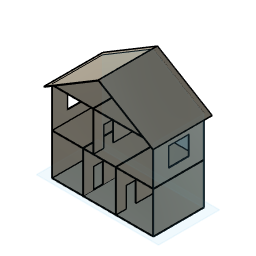
model (Autodesk Fusion 360 design; units mm, degrees)
Autodesk Fusion 360 part; units mm, degrees
note: some values were not read from the file. Set by a fixed rule: which sketch regions a step uses.
sketch "Sketch1" plane through (0, 0, 0) normal (0, 0, 1) x (1, 0, 0)
  line L0 (-300, 150) -> (300, 150)
  line L1 (300, 150) -> (300, -150)
  line L2 (300, -150) -> (-300, -150)
  line L3 (-300, -150) -> (-300, 150)
  line L4 (-300, 0) -> (300, 0) construction
  dimension "d4" = 600
  dimension "d5" = 300
  constraint horizontal L0
  constraint vertical L1
  constraint horizontal L2
  constraint vertical L3
  constraint midpoint L3 L4.start
  constraint midpoint L1 L4.end
  constraint midpoint origin L4
  measures "d4" distance of L0.start L0.end
  measures "d5" distance of L0.start L2.end
sketch "Sketch2" plane through (0, 0, 0) normal (0, 0, -1) x (1, 0, 0)
  line L0 (300, 150) -> (-300, 150)
  line L1 (-300, 150) -> (-300, -150)
  line L2 (-300, -150) -> (300, -150)
  line L3 (300, -150) -> (300, 150)
  line L4 (-250, 125) -> (-247, 125)
  line L5 (-247, 125) -> (-247, -125)
  line L6 (-247, -125) -> (-250, -125)
  line L7 (-250, -125) -> (-250, 125)
  line L8 (250, 125) -> (247, 125)
  line L9 (247, 125) -> (247, -125)
  line L10 (247, -125) -> (250, -125)
  line L11 (250, -125) -> (250, 125)
  dimension "d8" = 3
  dimension "d9" = 3
  dimension "d10" = 50
  dimension "d11" = 50
  dimension "d12" = 25
  dimension "d13" = 25
  dimension "d14" = 25
  dimension "d15" = 25
  constraint horizontal L4
  constraint vertical L5
  constraint horizontal L6
  constraint vertical L7
  constraint horizontal L8
  constraint vertical L9
  constraint horizontal L10
  constraint vertical L11
  measures "d8" distance of L5 L7
  measures "d9" distance of L9 L11
  measures "d10" distance of L3 L11
  measures "d11" distance of L1 L7
  measures "d12" distance of L0 L4.start
  measures "d13" distance of L0 L8.start
  measures "d14" distance of L2 L9.end
  measures "d15" distance of L2 L5.end
extrude "Extrude2" add sketch "Sketch2" against normal blind 400 contours L4 L5 L6 L7 | L8 L9 L10 L11 makes body 1 at (-247, -41.6667, 133.3333) makes body 2 at (250, 41.6667, 133.3333)
sketch "Sketch3" plane through (0, 0, 0) normal (0, 0, -1) x (1, 0, 0)
  line L0 (300, 150) -> (-300, 150)
  line L1 (-300, 150) -> (-300, -150)
  line L2 (-300, -150) -> (300, -150)
  line L3 (300, -150) -> (300, 150)
  line L4 (-250, -125) -> (-250, 125)
  line L5 (250, -125) -> (250, 125)
  line L6 (-250, -125) -> (250, -125)
  line L7 (250, -125) -> (250, -122)
  line L8 (250, -122) -> (-250, -122)
  line L9 (-250, -122) -> (-250, -125)
  dimension "d18" = 3
  constraint horizontal L6
  constraint vertical L7
  constraint horizontal L8
  constraint vertical L9
  constraint coincident L5 L7.end
  constraint coincident L4.start L6.start
  measures "d18" distance of L6 L8
extrude "Extrude3" add sketch "Sketch3" against normal blind 400 separate body contours L4 L5 L6 L7 L8 L9 makes body 3
sketch "Sketch4" plane through (0, 125, 0) normal (0, 1, 0) x (-1, 0, 0)
  line L0 (-250, 0) -> (250, 0)
  line L1 (250, 0) -> (250, 400)
  line L2 (250, 400) -> (-250, 400)
  line L3 (-250, 400) -> (-250, 0)
  line L4 (-250, 400) -> (0, 550)
  line L5 (0, 550) -> (250, 400)
  line L6 (0, 550) -> (0, 400) construction
  dimension "d21" = 150
  constraint coincident L2.end L3.start
  constraint coincident L1.end L2.start
  constraint midpoint L2 L6.end
  constraint perpendicular L2 L6
  measures "d21" distance of L4.end L6.end
extrude "Extrude4" add sketch "Sketch4" against normal blind 3 separate body contours L2 L4 L5 makes body 4
combine "Combine1" operation add target body 3 tool bodies 4
sketch "Sketch5" plane through (242.6471, 0, 404.4118) normal (0.514496, 0, 0.857493) x (0, 1, 0)
  line L0 (125, -8.5749) -> (125, 282.9727)
  line L1 (125, 282.9727) -> (122, 282.9727)
  line L2 (122, 282.9727) -> (122, -8.5749)
  line L3 (122, -8.5749) -> (125, -8.5749)
  line L4 (145, 285.9727) -> (-145, 285.9727)
  line L5 (-145, 285.9727) -> (-145, -28.5749)
  line L6 (-145, -28.5749) -> (145, -28.5749)
  line L7 (145, -28.5749) -> (145, 285.9727)
  line L8 (-125, -214.3732) -> (-125, -8.5749)
  line L9 (-125, -8.5749) -> (125, -8.5749)
  dimension "d24" = 20
  dimension "d25" = 20
  dimension "d26" = 3
  dimension "d27" = 20
  constraint horizontal L4
  constraint vertical L5
  constraint horizontal L6
  constraint vertical L7
  measures "d24" distance of L0 L6.end
  measures "d25" distance of L5 L8
  measures "d26" distance of L1.end L4
  measures "d27" distance of L6 L9
extrude "Extrude5" add sketch "Sketch5" along normal blind 3 separate body contours L0 L1 L2 L3 L9 | L4 L5 L6 L7 makes body 5
sketch "Sketch6" plane through (-242.6471, 0, 404.4118) normal (-0.514496, 0, 0.857493) x (0, -1, 0)
  line L0 (-125, 282.9727) -> (-125, -8.5749)
  line L1 (-125, -8.5749) -> (-122, -8.5749)
  line L2 (-122, -8.5749) -> (-122, 282.9727)
  line L3 (-122, 282.9727) -> (-125, 282.9727)
  line L4 (-145, 281.5609) -> (145, 281.5609)
  line L5 (-145, 281.5609) -> (145, 281.5609)
  line L6 (145, 281.5609) -> (145, -28.5749)
  line L7 (145, -28.5749) -> (-145, -28.5749)
  line L8 (-145, -28.5749) -> (-145, 281.5609)
  dimension "d30" = 20
  constraint horizontal L5
  constraint vertical L6
  constraint horizontal L7
  constraint vertical L8
  constraint coincident L4.start L5.start
  constraint vertical L4.end L6.end
  measures "d30" distance of L1.end L7
extrude "Extrude6" add sketch "Sketch6" along normal blind 3 contours L0 L1 L2 L4 L5 | L0 L1 L2 L4 L5 L6 L7 L8 bodies 1 3 5
sketch "Back wall" plane through (0, 122, 0) normal (0, -1, 0) x (1, 0, 0)
  line L0 (-250, 400) -> (-247, 400)
  line L1 (-247, 400) -> (-247, 0)
  line L2 (-247, 0) -> (250, 0)
  line L3 (250, 0) -> (250, 400)
  line L4 (250, 400) -> (0, 550)
  line L5 (0, 550) -> (-1.2106, 549.2737)
  line L6 (-1.2106, 549.2737) -> (-250, 400)
split "Split1" by plane through (-244.1905, 0, 406.9842) normal (-0.514496, 0, 0.857493) bodies 1 makes body 6 at (-1.8007, 48.3333, 552.8297)
delete_body "RemoveBody1" bodies 6
sketch "Sketch8" plane through (0, 0, 3) normal (0, 0, 1) x (-1, 0, 0)
  line L0 (300, 150) -> (-300, 150)
  line L1 (-300, 150) -> (-300, -150)
  line L2 (-300, -150) -> (300, -150)
  line L3 (300, -150) -> (300, 150)
ref_plane "WorkPlane2" through (0, 0, 203) normal (0, 0, 1) x (1, 0, 0)
sketch "Sketch9" plane through (0, 0, 203) normal (0, 0, 1) x (1, 0, 0)
ref_plane "WorkPlane3" through (0, 0, 203) normal (0, 0, 1) x (1, 0, 0)
sketch "2nd floor" plane through (0, 0, 203) normal (0, 0, 1) x (1, 0, 0)
  line L0 (-247, 122) -> (-247, -125)
  line L1 (-247, -125) -> (-247, 122)
  line L2 (-250, 122) -> (-247, 122)
  line L3 (-247, 122) -> (250, 122)
  line L4 (250, 122) -> (0, 122)
  line L5 (0, 122) -> (-1.2106, 122)
  line L6 (-1.2106, 122) -> (-250, 122)
  line L7 (250, -125) -> (250, 125)
  line L8 (250, 125) -> (250, -125)
  line L9 (-247, 122) -> (250, 122)
  line L10 (250, 122) -> (250, -125)
  line L11 (250, -125) -> (-247, -125)
  line L12 (-247, -125) -> (-247, 122)
  constraint horizontal L9
  constraint vertical L10
  constraint horizontal L11
  constraint vertical L12
  constraint coincident L7.start L8.end
  constraint coincident L0.start L1.end
extrude "Extrude7" add sketch "2nd floor" along normal blind 3 separate body makes body 7
ref_plane "WorkPlane4" through (0, 0, 400) normal (0, 0, 1) x (-1, 0, 0)
sketch "Sketch11" plane through (0, 0, 400) normal (0, 0, 1) x (1, 0, 0)
  line L0 (-247, 122) -> (-247, -125)
  line L1 (-247, -125) -> (-247, 122)
  line L2 (-250, 122) -> (-247, 122)
  line L3 (-247, 122) -> (250, 122)
  line L4 (250, 122) -> (0, 122)
  line L5 (0, 122) -> (-1.2106, 122)
  line L6 (-1.2106, 122) -> (-250, 122)
  line L7 (250, -125) -> (250, 125)
  line L8 (250, 125) -> (250, -125)
  line L9 (-247, 122) -> (250, 122)
  line L10 (250, 122) -> (250, -125)
  line L11 (250, -125) -> (-247, -125)
  line L12 (-247, -125) -> (-247, 122)
  constraint horizontal L9
  constraint vertical L10
  constraint horizontal L11
  constraint vertical L12
  constraint coincident L7.start L8.end
  constraint coincident L0.start L1.end
extrude "Extrude8" add sketch "Sketch11" against normal blind 3 separate body makes body 8
ref_plane "WorkPlane5" through (-97, -1.5, 200) normal (1, 0, 0) x (0, 1, 0)
sketch "Sketch12" plane through (-97, 0, 0) normal (1, 0, 0) x (0, 1, 0)
  line L0 (122, 400) -> (122, 0)
  line L1 (122, 0) -> (122, 400)
  line L2 (122, 400) -> (122, 550)
  line L3 (122, 550) -> (122, 549.2737)
  line L4 (122, 549.2737) -> (122, 400)
  line L5 (125, 0) -> (-125, 0)
  line L6 (-125, 0) -> (-125, 400)
  line L7 (-125, 400) -> (122, 400)
  line L8 (122, 400) -> (125, 400)
  line L9 (125, 400) -> (125, 0)
  line L10 (-125, 206) -> (122, 206)
  line L11 (122, 206) -> (-125, 206)
  line L12 (125, 0) -> (125, 400)
  line L13 (125, 400) -> (125, 549.2737)
  line L14 (125, 549.2737) -> (125, 550)
  line L15 (125, 550) -> (125, 400)
  line L16 (125, 400) -> (125, 0)
  line L17 (-125, 400) -> (122, 400)
  line L18 (122, 400) -> (122, 206)
  line L19 (122, 206) -> (-125, 206)
  line L20 (-125, 206) -> (-125, 400)
  point P0 (-125, 400)
  constraint horizontal L17
  constraint vertical L18
  constraint horizontal L19
  constraint vertical L20
  constraint coincident L10.end L11.start
  constraint coincident P0 L6.end
extrude "Extrude9" add sketch "Sketch12" along normal blind 3 separate body contours L0 L1 L6 L7 L10 L11 L17 L18 L19 L20 makes body 9
ref_plane "WorkPlane6" through (67, 0, 200) normal (-1, 0, 0) x (0, -1, 0)
sketch "Sketch13" plane through (67, 0, 0) normal (-1, 0, 0) x (0, -1, 0)
  line L0 (-122, 400) -> (-122, 0)
  line L1 (-122, 0) -> (-122, 400)
  line L2 (-122, 400) -> (-122, 550)
  line L3 (-122, 550) -> (-122, 549.2737)
  line L4 (-122, 549.2737) -> (-122, 400)
  line L5 (150, 3) -> (-150, 3)
  line L6 (-150, 3) -> (150, 3)
  line L7 (125, 206) -> (-122, 206)
  line L8 (-122, 206) -> (-122, 0)
  line L9 (-122, 0) -> (125, 0)
  line L10 (125, 0) -> (125, 206)
  point P0 (125, 206)
  constraint horizontal L7
  constraint vertical L8
  constraint horizontal L9
  constraint vertical L10
  constraint coincident L0.end L1.start
  constraint coincident P0 L7.start
extrude "Extrude10" add sketch "Sketch13" along normal blind 3 separate body contours L0 L1 L5 L6 L7 L8 L10 makes body 10
ref_plane "WorkPlane7" through (-97, -1.5, 200) normal (1, 0, 0) x (0, 1, 0)
sketch "Sketch14" plane through (-97, 0, 0) normal (1, 0, 0) x (0, 1, 0)
  line L0 (122, 400) -> (122, 0)
  line L1 (122, 0) -> (122, 400)
  line L2 (122, 400) -> (122, 550)
  line L3 (122, 550) -> (122, 549.2737)
  line L4 (122, 549.2737) -> (122, 400)
  line L5 (-125, 206) -> (122, 206)
  line L6 (122, 206) -> (122, 0)
  line L7 (122, 0) -> (-125, 0)
  line L8 (-125, 0) -> (-125, 206)
  point P0 (-125, 206)
  point P1 (122, 0)
  constraint horizontal L5
  constraint vertical L6
  constraint horizontal L7
  constraint vertical L8
  constraint coincident P1 L0.end
  constraint coincident P0 L5.start
extrude "Extrude11" add sketch "Sketch14" along normal blind 3 separate body makes body 11
sketch "Sketch15" plane through (0, 122, 0) normal (0, -1, 0) x (1, 0, 0)
  line L0 (-250, 400) -> (-247, 400)
  line L1 (-247, 400) -> (-247, 0)
  line L2 (-247, 0) -> (250, 0)
  line L3 (250, 0) -> (250, 400)
  line L4 (250, 400) -> (0, 550)
  line L5 (0, 550) -> (-1.2106, 549.2737)
  line L6 (-1.2106, 549.2737) -> (-250, 400)
move_body "Move1" bodies 9 to x (1, 0, 0) y (0, 1, 0) z (0, 0, 1) at (50, 0, 0)
sketch "Sketch16" plane through (-44, 0, 0) normal (1, 0, 0) x (0, 1, 0)
  line L0 (-125, 206) -> (122, 206)
  line L1 (122, 206) -> (122, 400)
  line L2 (122, 400) -> (-125, 400)
  line L3 (-125, 400) -> (-125, 206)
  line L4 (-75, 206) -> (-28, 206)
  line L5 (-28, 206) -> (-28, 306)
  line L6 (-28, 306) -> (-75, 306)
  line L7 (-75, 306) -> (-75, 206)
  dimension "d50" = 50
  dimension "d51" = 150
  dimension "d52" = 100
  constraint horizontal L4
  constraint vertical L5
  constraint horizontal L6
  constraint vertical L7
  constraint coincident L0 L4.start
  measures "d50" distance of L3 L7
  measures "d51" distance of L1 L5
  measures "d52" distance of L4 L6
extrude "Extrude12" cut sketch "Sketch16" against normal blind 3 contours L0 L4 L5 L6 L7 bodies 9
sketch "Sketch17" plane through (67, 0, 0) normal (1, 0, 0) x (0, 1, 0)
  line L0 (-125, 3) -> (122, 3)
  line L1 (122, 3) -> (122, 206)
  line L2 (122, 206) -> (-125, 206)
  line L3 (-125, 206) -> (-125, 3)
  line L4 (122, 3) -> (-125, 3)
  line L5 (-75, 3) -> (-28, 3)
  line L6 (-28, 3) -> (-28, 103)
  line L7 (-28, 103) -> (-75, 103)
  line L8 (-75, 103) -> (-75, 3)
  dimension "d55" = 50
  dimension "d56" = 150
  dimension "d57" = 100
  constraint horizontal L5
  constraint vertical L6
  constraint horizontal L7
  constraint vertical L8
  constraint coincident L0 L5.start
  measures "d55" distance of L3 L8
  measures "d56" distance of L1 L6
  measures "d57" distance of L5 L7
extrude "Extrude13" cut sketch "Sketch17" against normal blind 3 contours L0 L4 L5 L6 L7 L8 bodies 10
sketch "Sketch18" plane through (-94, 0, 0) normal (1, 0, 0) x (0, 1, 0)
  line L0 (-125, 0) -> (122, 0)
  line L1 (122, 0) -> (122, 206)
  line L2 (122, 206) -> (-125, 206)
  line L3 (-125, 206) -> (-125, 0)
  line L4 (-150, 3) -> (150, 3)
  line L5 (150, 3) -> (-150, 3)
  line L6 (-75, 3) -> (-28, 3)
  line L7 (-28, 3) -> (-28, 103)
  line L8 (-28, 103) -> (-75, 103)
  line L9 (-75, 103) -> (-75, 3)
  dimension "d60" = 50
  dimension "d61" = 100
  dimension "d62" = 150
  constraint horizontal L6
  constraint vertical L7
  constraint horizontal L8
  constraint vertical L9
  constraint coincident L5 L6.start
  measures "d60" distance of L3 L9
  measures "d61" distance of L6 L8
  measures "d62" distance of L1 L7
extrude "Extrude14" cut sketch "Sketch18" against normal blind 3 contours L4 L5 L6 L7 L8 L9 bodies 11
sketch "Sketch19" plane through (0, 0, 3) normal (0, 0, 1) x (-1, 0, 0)
  line L0 (247, -122) -> (247, 125)
  line L1 (247, 125) -> (247, -122)
  line L2 (250, -122) -> (247, -122)
  line L3 (247, -122) -> (-250, -122)
  line L4 (-250, -122) -> (0, -122)
  line L5 (0, -122) -> (1.2106, -122)
  line L6 (1.2106, -122) -> (250, -122)
  line L7 (-250, 125) -> (-250, -125)
  line L8 (-250, -125) -> (-250, 125)
  line L9 (250, -122) -> (-250, -122)
  line L10 (-250, -122) -> (-250, 125)
  line L11 (-250, 125) -> (250, 125)
  line L12 (250, 125) -> (250, -122)
  line L13 (250, -122) -> (-250, -122)
  line L14 (-250, -122) -> (-250, -125)
  line L15 (-250, -125) -> (250, -125)
  line L16 (250, -125) -> (250, -122)
  line L17 (250, -122) -> (-250, -122)
  line L18 (-250, -122) -> (-250, 125)
  line L19 (-250, 125) -> (250, 125)
  line L20 (250, 125) -> (250, -122)
  constraint horizontal L9
  constraint vertical L10
  constraint horizontal L11
  constraint vertical L12
  constraint coincident L7.start L8.end
  constraint coincident L2.start L6.end
  constraint horizontal L13
  constraint vertical L14
  constraint horizontal L15
  constraint vertical L16
  constraint coincident L7.end L8.start
  constraint horizontal L17
  constraint vertical L18
  constraint horizontal L19
  constraint vertical L20
extrude "Extrude15" add sketch "Sketch19" against normal blind 3 separate body contours L0 L1 L3 L4 L5 L6 L7 L8 L9 L10 L11 L13 L17 L18 L19 makes body 12
sketch "Sketch20" plane through (-247, 0, 0) normal (1, 0, 0) x (0, 1, 0)
  line L0 (122, 0) -> (122, 400)
  line L1 (122, 400) -> (-125, 400)
  line L2 (-125, 400) -> (-125, 0)
  line L3 (-125, 0) -> (122, 0)
  line L4 (-50, 347) -> (47, 347)
  line L5 (47, 347) -> (47, 256)
  line L6 (47, 256) -> (-50, 256)
  line L7 (-50, 256) -> (-50, 347)
  line L8 (122, 206) -> (-125, 206)
  line L9 (-125, 397) -> (122, 397)
  dimension "d67" = 75
  dimension "d68" = 50
  dimension "d69" = 75
  dimension "d70" = 50
  constraint horizontal L4
  constraint vertical L5
  constraint horizontal L6
  constraint vertical L7
  measures "d67" distance of L2 L7
  measures "d68" distance of L6 L8
  measures "d69" distance of L0 L5
  measures "d70" distance of L4 L9
extrude "Extrude16" cut sketch "Sketch20" against normal blind 3 contours L4 L5 L6 L7 bodies 1
sketch "Sketch21" plane through (250, 0, 0) normal (1, 0, 0) x (0, 1, 0)
  line L0 (-125, 0) -> (125, 0)
  line L1 (125, 0) -> (125, 400)
  line L2 (125, 400) -> (-125, 400)
  line L3 (-125, 400) -> (-125, 0)
  line L4 (-50, 350) -> (50, 350)
  line L5 (50, 350) -> (50, 256)
  line L6 (50, 256) -> (-50, 256)
  line L7 (-50, 256) -> (-50, 350)
  line L8 (-50, 153) -> (50, 153)
  line L9 (50, 153) -> (50, 53)
  line L10 (50, 53) -> (-50, 53)
  line L11 (-50, 53) -> (-50, 153)
  line L12 (-150, 3) -> (150, 3)
  line L13 (-125, 206) -> (122, 206)
  point P0 (0, 203)
  dimension "d73" = 75
  dimension "d74" = 75
  dimension "d75" = 50
  dimension "d76" = 50
  dimension "d77" = 75
  dimension "d78" = 75
  dimension "d79" = 50
  dimension "d80" = 50
  constraint horizontal L4
  constraint vertical L5
  constraint horizontal L6
  constraint vertical L7
  constraint horizontal L8
  constraint vertical L9
  constraint horizontal L10
  constraint vertical L11
  measures "d73" distance of L3 L11
  measures "d74" distance of L1 L9
  measures "d75" distance of L8 P0
  measures "d76" distance of L10 L12
  measures "d77" distance of L1 L5
  measures "d78" distance of L3 L7
  measures "d79" distance of L2 L4
  measures "d80" distance of L6 L13
extrude "Extrude17" cut sketch "Sketch21" against normal blind 3 contours L4 L5 L6 L7 bodies 2
sketch "Sketch22" plane through (250, 0, 0) normal (1, 0, 0) x (0, 1, 0)
  line L0 (50, 350) -> (50, 256)
  line L1 (50, 256) -> (-50, 256)
  line L2 (-50, 256) -> (-50, 350)
  line L3 (-50, 350) -> (50, 350)
  line L4 (-125, 0) -> (125, 0)
  line L5 (125, 0) -> (125, 400)
  line L6 (125, 400) -> (-125, 400)
  line L7 (-125, 400) -> (-125, 0)
equation "Walls = 3 mm"
equation "Base = 3 mm"
equation "Trim = 3 mm"
equation "d8 = Walls"
equation "d9 = Walls"
equation "d18 = Walls"
equation "d22 = -Walls"
equation "d26 = Walls"
equation "d28 = Walls"
equation "d31 = Walls"
equation "All = 3 mm"
equation "d53 = -Walls"
named bodies: "Left wall", "Right wall", "Back wall", "Right roof", "Left wall (", "2nd floor", "inside roof", "1. Floor wall", "1. Floor wall2"
